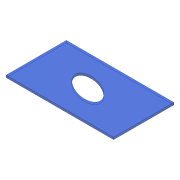
# Autodesk Inventor part: ThickThinProfile
Saved by Autodesk Inventor 2014 (Build 180170000, 170)
## iProperties
Created: 2014-12-16
Part Number: ThickThinProfile
Material: Generic
Document SubType Name: Sheet Metal
Designer: Yogesh
Density: 1 g/cm^3
Appearance: Clear - Blue
Sheet Metal Rule: Default
Author: Yogesh
Autodesk Inventor part; units mm, degrees
ref_plane "YZ Plane" through (0, 0, 0) normal (1, 0, 0) x (0, 1, 0)
ref_plane "XZ Plane" through (0, 0, 0) normal (0, 1, 0) x (-1, 0, 0)
ref_plane "XY Plane" through (0, 0, 0) normal (0, 0, 1) x (1, 0, 0)
sketch "Sketch2" plane through (0, 0, 0) normal (0, 0, 1) x (1, 0, 0)
  line L0 (0, 0) -> (25, 0)
  line L1 (25, 0) -> (25, 14)
  line L2 (25, 14) -> (0, 14)
  line L3 (0, 14) -> (0, 0)
extrude "Plate1" add sketch "Sketch2" along normal blind 0.5
sketch "Sketch3" plane through (0, 0, 0.5) normal (0, 0, 1) x (1, 0, 0)
  ellipse E0 centre (12, 7) end of major axis (7.9562, 8.7331) minor radius 2.2351
  constraints: 2 other
extrude "Cut1" cut sketch "Sketch3" against normal blind 0.5
equation "\"d5\" = Thickness"
equation "\"BendRadius\" = Thickness"
equation "\"BendReliefWidth\" = Thickness"
equation "\"BendReliefDepth\" = 0.5 * Thickness"
equation "\"CornerReliefSize\" = 4 * Thickness"
equation "\"MinimumRemnant\" = 2 * Thickness"
equation "\"TransitionRadius\" = BendRadius"
equation "\"JacobiRadiusSize\" = Thickness"
equation "\"GapSize\" = Thickness"
equation "\"d4\" = BendRadius"
equation "\"Thickness\" = 0.5"
body "Solid2"
